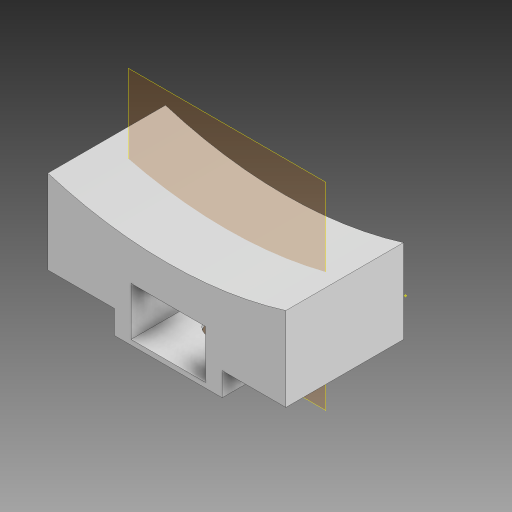
# Autodesk Inventor part: kicker1.1
Saved by Autodesk Inventor 2023 (Build 270158000, 158)
## iProperties
Created: 2025-04-11
Part Number: kicker1.1
Material: Типовые
Document SubType Name: Modeling
Designer: Ivan
Density: 1 g/cm^3
Appearance: По умолчанию
Author: Ivan
Autodesk Inventor part; units mm, degrees
ref_plane "YZ Plane" through (0, 0, 0) normal (1, 0, 0) x (0, 1, 0)
ref_plane "XZ Plane" through (0, 0, 0) normal (0, 1, 0) x (-1, 0, 0)
ref_plane "XY Plane" through (0, 0, 0) normal (0, 0, 1) x (1, 0, 0)
ref_plane "РабПлоскость2" through (19.838, 4.4675, -12.3) normal (0, 0, 1) x (1, 0, 0)
ref_plane "РабПлоскость1" through (-13.412, 18.3334, -19.05) normal (0, 0, 1) x (1, 0, 0)
sketch "Эскиз1" plane through (19.838, 4.4675, -12.3) normal (0, 0, 1) x (1, 0, 0)
  line L0 (-17.838, -7.8158) -> (-21.838, -7.8158) projected
  line L1 (-21.838, -12.9158) -> (-17.838, -12.9158) projected
  line L2 (-15.838, -12.5585) -> (-15.838, -8.173) projected
  line L3 (-23.838, -12.5585) -> (-23.838, -8.173) projected
  line L4 (-15.688, -12.9158) -> (-23.988, -12.9158)
  line L5 (-23.988, -12.9158) -> (-23.988, -7.5158)
  line L6 (-23.988, -7.5158) -> (-15.688, -7.5158)
  line L7 (-15.688, -7.5158) -> (-15.688, -12.9158)
  line L8 (-15.688, -12.9158) -> (-23.988, -7.5158) construction
  line L9 (-19.838, -4.4675) -> (-19.838, -10.2158) construction
  line L10 (-15.388, -12.9158) -> (-24.288, -12.9158)
  line L11 (-6.75, -10.8528) -> (-33.25, -10.8528) projected
  line L12 (-33.25, -10.8528) -> (-6.75, -10.8528) projected
  line L13 (-33.25, -10.8528) -> (-6.75, -10.8528) construction
  line L14 (-24.938, -14.0158) -> (-14.738, -14.0158) projected
  line L15 (-15.388, -12.9158) -> (-24.288, -12.9158)
  line L16 (-19.838, -14.0158) -> (-19.838, -12.9158) construction
  line L17 (-13.838, -13.4658) -> (-25.838, -13.4658) construction
  line L18 (-25.838, -13.4658) -> (-25.838, -3.5158)
  line L19 (-25.838, -3.5158) -> (-13.838, -3.5158)
  line L20 (-13.838, -3.5158) -> (-13.838, -13.4658)
  line L21 (-6.75, -10.8528) -> (-33.25, -10.8528)
  line L22 (-33.25, -10.8528) -> (-33.25, -3.5158)
  line L23 (-33.25, -3.5158) -> (-6.75, -3.5158)
  line L24 (-6.75, -3.5158) -> (-6.75, -10.8528)
  line L25 (-6.75, -3.5158) -> (-6.75, -1.5158)
  line L26 (-33.25, -3.5158) -> (-33.25, -1.5158)
  arc A0 (-33.25, -1.5158) -> (-6.75, -1.5158) centre (-20, 41.3683) ccw
  line L27 (-25.838, -13.4658) -> (-13.838, -13.4658) construction
  line L28 (-13.838, -13.4658) -> (-13.838, -13.4658)
  line L29 (-13.838, -13.4658) -> (-25.838, -13.4658)
  line L30 (-25.838, -13.4658) -> (-25.838, -13.4658)
  point P0 (-19.838, -13.4658)
  point P1 (-19.838, -3.5158)
  point P2 (-25.838, -10.8528)
  point P3 (-13.838, -10.8528)
  point P4 (-20.162, -3.5158)
  point P5 (-15.688, -10.8528)
  point P6 (-23.988, -10.8528)
  dimension "d0" = 8.3
  dimension "d1" = 5.4
  dimension "d2" = 12
  dimension "d3" = 4
  dimension "d4" = 2
  dimension "d10" = 0
  dimension "d11" = 0.55
  constraints: 46 end point, 8 equal length, 7 midpoint, 6 horizontal, 4 perpendicular, 4 vertical, 3 point on circle, 2 point on line, 1 centre point, 1 parallel, 2 other
  measures "d0" distance between parallel lines of L5 L7
  measures "d1" distance between parallel lines of L4 L6
  measures "d2" distance between parallel lines of L20 L18
  measures "d3" distance from line of L6 point (-19.838, -3.516)
  measures "d4" distance of L22.end L26.end
  measures "d10" distance of L27.end L28.end
  measures "d11" distance between parallel lines of L4 L29
extrude "Выдавливание1" add sketch "Эскиз1" along normal mid plane 13.1 contours L1 L4 L7 L11 L20 L29 L18 L5 | L11 L18 L19 L20 L7 L6 L5 | L11 L22 L23 L18 | L20 L23 L24 L11 | L23 L26 A0 L19 | L19 A0 L25 L23
sketch "Эскиз3" plane through (-6, -8.9982, -5.75) normal (0, -1, 0) x (1, 0, 0)
  line L0 (-7.412, 0) -> (0, 0) projected
  line L1 (12, -13.1) -> (12, 0) projected
  line L2 (0, 0) -> (12, -13.1) construction
  circle A0 centre (6, -6.55) radius 2
  point P0 (6, 5.75)
  dimension "d12" = 4
  constraints: 2 end point, 1 centre point, 1 midpoint
  measures "d12" diameter of A0
extrude "Выдавливание3" cut sketch "Эскиз3" against normal up to surface (5.95 mm away)
